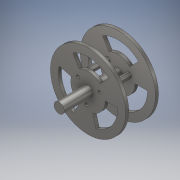
# Autodesk Inventor part: platform_wheel
Saved by Autodesk Inventor 2019 (Build 230136000, 136)
## iProperties
Created: 2020-06-10
Part Number: platform_wheel
Material: Generic
Document SubType Name: Modeling
Designer: Jorge
Density: 1 g/cm^3
Appearance: Default
Author: Jorge
Autodesk Inventor part; units mm, degrees
ref_plane "YZ Plane" through (0, 0, 0) normal (1, 0, 0) x (0, 1, 0)
ref_plane "XZ Plane" through (0, 0, 0) normal (0, 1, 0) x (-1, 0, 0)
ref_plane "XY Plane" through (0, 0, 0) normal (0, 0, 1) x (1, 0, 0)
sketch "Sketch1" plane through (0, 0, 0) normal (0, 0, 1) x (1, 0, 0)
  circle A0 centre (0, 0) radius 24
  circle A1 centre (0, 0) radius 3.5
  arc A2 (7.6927, 7.8627) -> (-5.6038, 9.4656) centre (0, 0) ccw
  line L0 (0, 0) -> (7.6927, 7.8627) construction
  line L1 (0, 0) -> (-5.6038, 9.4656) construction
  arc A3 (13.2874, 13.5811) -> (-9.6793, 16.3497) centre (0, 0) ccw
  line L2 (0, 0) -> (13.2874, 13.5811) construction
  line L3 (0, 0) -> (-9.6793, 16.3497) construction
  line L4 (-5.6038, 9.4656) -> (-9.6793, 16.3497)
  line L5 (7.6927, 7.8627) -> (13.2874, 13.5811)
  arc A4 (5.1178, -18.2977) -> (18.9989, 0.2077) centre (0, 0) ccw
  line L6 (0, 0) -> (18.9989, 0.2077) construction
  line L7 (10.9993, 0.1202) -> (18.9989, 0.2077)
  line L8 (0, 0) -> (5.1178, -18.2977) construction
  line L9 (2.963, -10.5934) -> (5.1178, -18.2977)
  arc A5 (2.963, -10.5934) -> (10.9993, 0.1202) centre (0, 0) ccw
  arc A6 (-18.4052, 4.7167) -> (-9.3196, -16.5573) centre (0, 0) ccw
  line L10 (0, 0) -> (-9.3196, -16.5573) construction
  line L11 (-5.3956, -9.5858) -> (-9.3196, -16.5573)
  line L12 (0, 0) -> (-18.4052, 4.7167) construction
  line L13 (-10.6557, 2.7307) -> (-18.4052, 4.7167)
  arc A7 (-10.6557, 2.7307) -> (-5.3956, -9.5858) centre (0, 0) ccw
  circle A8 centre (-6.3997, 4.8004) radius 1
  line L14 (-6.3997, 4.8004) -> (0, 0) construction
  circle A9 centre (-0.9575, -7.9425) radius 1
  circle A10 centre (7.3571, 3.1421) radius 1
  dimension "d0" = 48
  dimension "d1" = 7
  dimension "d2" = 11
  dimension "a1" = 75
  dimension "d4" = 19
  dimension "d5" = 75
  dimension "d8" = 360
  dimension "d10" = 2
  dimension "d11" = 8
  dimension "d12" = 22.5
  dimension "d15" = 360
  constraints: 30 end point, 12 point on circle, 11 centre point, 6 coincident, 1 collinear, 44 other
  measures "d0" diameter of A0
  measures "d1" diameter of A1
  measures "d2" radius of A2
  measures "a1" angle of L0 L1
  measures "d4" radius of A3
  measures "d5" angle of L2 L3
  measures "d10" diameter of A8
  measures "d11" distance of L14.start L14.end
  measures "d12" angle of L1 L14
extrude "Extrusion1" add sketch "Sketch1" along normal blind 2
extrude "Extrusion2" add sketch "Sketch1" along normal blind 21 contours A1
sketch "Sketch2" plane through (0, 0, 21) normal (0, 0, 1) x (1, 0, 0)
  line L0 (-18.4052, 4.7167) -> (-10.6557, 2.7307) projected
  arc A0 (-10.6557, 2.7307) -> (-5.3956, -9.5858) centre (0, 0) ccw projected
  line L1 (-5.3956, -9.5858) -> (-9.3196, -16.5573) projected
  arc A1 (-18.4052, 4.7167) -> (-9.3196, -16.5573) centre (0, 0) ccw projected
  line L2 (5.1178, -18.2977) -> (2.963, -10.5934) projected
  arc A2 (2.963, -10.5934) -> (10.9993, 0.1202) centre (0, 0) ccw projected
  line L3 (10.9993, 0.1202) -> (18.9989, 0.2077) projected
  arc A3 (5.1178, -18.2977) -> (18.9989, 0.2077) centre (0, 0) ccw projected
  line L4 (-5.6038, 9.4656) -> (-9.6793, 16.3497) projected
  arc A4 (13.2874, 13.5811) -> (-9.6793, 16.3497) centre (0, 0) ccw projected
  line L5 (13.2874, 13.5811) -> (7.6927, 7.8627) projected
  arc A5 (7.6927, 7.8627) -> (-5.6038, 9.4656) centre (0, 0) ccw projected
  circle A6 centre (0, 0) radius 3.5 projected
  circle A7 centre (7.3571, 3.1421) radius 1 projected
  circle A8 centre (-0.9575, -7.9425) radius 1 projected
  circle A9 centre (-6.3997, 4.8004) radius 1 projected
  circle A10 centre (0, 0) radius 24 projected
extrude "Extrusion3" add sketch "Sketch2" against normal blind 2
sketch "Sketch3" plane through (0, 0, 19) normal (0, 0, -1) x (-1, 0, 0)
  circle A0 centre (0, 0) radius 24 projected
  circle A1 centre (-7.3571, 3.1421) radius 1 projected
  circle A2 centre (0.9575, -7.9425) radius 1 projected
  circle A3 centre (6.3997, 4.8004) radius 1 projected
  arc A4 (9.3196, -16.5573) -> (18.4052, 4.7167) centre (0, 0) ccw projected
  line L0 (18.4052, 4.7167) -> (10.6557, 2.7307) projected
  arc A5 (5.3956, -9.5858) -> (10.6557, 2.7307) centre (0, 0) ccw projected
  line L1 (5.3956, -9.5858) -> (9.3196, -16.5573) projected
  arc A6 (-18.9989, 0.2077) -> (-5.1178, -18.2977) centre (0, 0) ccw projected
  line L2 (-5.1178, -18.2977) -> (-2.963, -10.5934) projected
  arc A7 (-10.9993, 0.1202) -> (-2.963, -10.5934) centre (0, 0) ccw projected
  line L3 (-10.9993, 0.1202) -> (-18.9989, 0.2077) projected
  arc A8 (5.6038, 9.4656) -> (-7.6927, 7.8627) centre (0, 0) ccw projected
  line L4 (5.6038, 9.4656) -> (9.6793, 16.3497) projected
  arc A9 (9.6793, 16.3497) -> (-13.2874, 13.5811) centre (0, 0) ccw projected
  line L5 (-13.2874, 13.5811) -> (-7.6927, 7.8627) projected
  circle A10 centre (0.9575, -7.9425) radius 1 projected
  line L6 (-0.6354, -7.2622) -> (0.7502, -6.2229)
  line L7 (0.7502, -6.2229) -> (2.343, -6.9032)
  line L8 (2.343, -6.9032) -> (2.5503, -8.6228)
  line L9 (2.5503, -8.6228) -> (1.1648, -9.6621)
  line L10 (1.1648, -9.6621) -> (-0.4281, -8.9818)
  line L11 (-0.4281, -8.9818) -> (-0.6354, -7.2622)
  line L12 (0, 0) -> (0.9575, -7.9425) construction
  line L13 (0, 0) -> (6.3997, 4.8004) construction
  line L14 (7.9925, 4.1202) -> (6.607, 3.0808)
  line L15 (6.607, 3.0808) -> (5.0141, 3.7611)
  line L16 (5.0141, 3.7611) -> (4.8068, 5.4807)
  line L17 (7.7852, 5.8398) -> (7.9925, 4.1202)
  line L18 (4.8068, 5.4807) -> (6.1924, 6.52)
  line L19 (6.1924, 6.52) -> (7.7852, 5.8398)
  line L20 (0, 0) -> (-7.3571, 3.1421) construction
  line L21 (-7.5644, 4.8617) -> (-5.9716, 4.1814)
  line L22 (-5.9716, 4.1814) -> (-5.7643, 2.4618)
  line L23 (-5.7643, 2.4618) -> (-7.1498, 1.4225)
  line L24 (-8.95, 3.8223) -> (-7.5644, 4.8617)
  line L25 (-7.1498, 1.4225) -> (-8.7427, 2.1027)
  line L26 (-8.7427, 2.1027) -> (-8.95, 3.8223)
  dimension "d23" = 3
  dimension "d26" = 360
  constraints: 42 end point, 3 coincident, 3 point on line, 65 other
  measures "d23" distance between parallel lines of L11 L8
extrude "Extrusion4" add sketch "Sketch3" along normal blind 17 contours L6 L7 L8 L9 L10 L11 | L14 L15 L16 L18 L19 L17 | L21 L22 L23 L25 L26 L24
sketch "Sketch4" plane through (0, 0, 21) normal (0, 0, 1) x (1, 0, 0)
  circle A0 centre (0, 0) radius 3.25
  dimension "d30" = 6.5
  constraints: 1 centre point, 1 coincident
  measures "d30" diameter of A0
extrude "Extrusion5" add sketch "Sketch4" along normal blind 18.5
equation "\"d5\" = a1"
body "Solid1"
